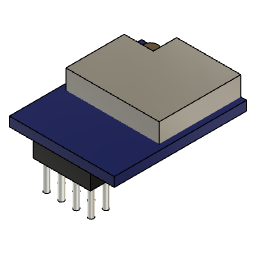
MLE21 v1.0 (Autodesk Fusion 360 archive; units mm, degrees)
design "RA-02"
Autodesk Fusion 360 part; units mm, degrees
sketch "Esquisse1" plane through (0, 0, 0) normal (0, 0, 1) x (1, 0, 0) in component "LoRa RA-02"
  line L0 (0, 0) -> (18, 0)
  line L1 (18, 0) -> (18, -22.7)
  line L2 (18, -22.7) -> (0, -22.7)
  line L3 (0, -22.7) -> (0, 0)
  line L4 (1, 0) -> (17, 0)
  line L5 (17, 0) -> (17, -14)
  line L6 (17, -14) -> (1, -14)
  line L7 (1, -14) -> (1, 0)
  line L8 (13.9, -22.7) -> (4.1, -22.7)
  line L9 (4.1, -22.7) -> (4.1, -17.7)
  line L10 (4.1, -17.7) -> (13.9, -17.7)
  line L11 (13.9, -17.7) -> (13.9, -22.7)
  line L12 (1, 0) -> (6, 0)
  line L13 (6, 0) -> (6, -4)
  line L14 (6, -4) -> (1, -4)
  line L15 (1, -4) -> (1, 0)
  circle A0 centre (3.5142, -2) radius 1.25
  circle A1 centre (5.2, -21.5) radius 0.445
  circle A2 centre (7.74, -21.5) radius 0.445
  circle A3 centre (10.28, -21.5) radius 0.445
  circle A4 centre (12.82, -21.5) radius 0.445
  circle A5 centre (5.2, -18.96) radius 0.445
  circle A6 centre (7.74, -18.96) radius 0.445
  circle A7 centre (10.28, -18.96) radius 0.445
  circle A8 centre (12.82, -18.96) radius 0.445
  dimension "d1" = 18
  dimension "d2" = 22.7
  dimension "d3" = 16
  dimension "d4" = 14
  dimension "d5" = 9.8
  dimension "d6" = 5
  dimension "d7" = 5
  dimension "d8" = 4
  dimension "d9" = 2.5
  dimension "d18" = 0.89
  dimension "d21" = 7.62
  dimension "d22" = 2.54
  dimension "d23" = 1.2
  dimension "d24" = 1.1
  constraint horizontal L0
  constraint vertical L1
  constraint horizontal L2
  constraint vertical L3
  constraint coincident L0.start L3.end
  constraint horizontal L4
  constraint vertical L5
  constraint horizontal L6
  constraint vertical L7
  constraint coincident L0 L4.start
  constraint midpoint L0 L4
  constraint horizontal L8
  constraint vertical L9
  constraint horizontal L10
  constraint vertical L11
  constraint coincident L2 L8.start
  constraint midpoint L2 L8
  constraint horizontal L12
  constraint vertical L13
  constraint horizontal L14
  constraint vertical L15
  measures "d1" distance of L0.start L0.end
  measures "d2" distance of L0.start L2.end
  measures "d3" distance of L4.start L4.end
  measures "d4" distance of L4.start L6.end
  measures "d5" distance of L8.start L8.end
  measures "d6" distance of L8.start L10.end
  measures "d7" distance of L4.start L12.end
  measures "d8" distance of L4.start L14.end
  measures "d9" diameter of A0
  measures "d18" diameter of A1
  measures "d23" distance of L2 A1.centre
  measures "d24" distance of L9 A1.centre
extrude "Extrusion1" add sketch "Esquisse1" along normal blind 1.6 contours L0 L1 L2 L3 L5 L6 L7 L9 L10 L11 L15 | L0 L4 L7 L12 L13 L14 L15 | L0 L4 L5 L6 L7 L13 L14 | L2 L8 L9 L10 L11 | A0 | A1 | A2 | A3 | A4 | A5 | A6 | A7 | A8 makes body 1 in component "LoRa RA-02"
extrude "Extrusion2" add sketch "Esquisse1" against normal blind 2.6 separate body contours L2 L8 L9 L10 L11 | A1 | A2 | A3 | A4 | A5 | A6 | A7 | A8 makes body 2 in component "LoRa RA-02"
extrude "Extrusion3" add sketch "Esquisse1" along normal blind 4.9 separate body contours L0 L4 L5 L6 L7 L13 L14 makes body 3 in component "LoRa RA-02"
extrude "Extrusion4" add sketch "Esquisse1" along normal blind 3 separate body contours A0 makes body 4 in component "LoRa RA-02"
extrude "Extrusion5" add sketch "Esquisse1" against normal blind 5 from surface at -2.6 separate body contours A1 | A2 | A3 | A4 | A5 | A6 | A7 | A8 makes body 5 at (10.077, -19.356, -4.2667) makes body 6 at (8.1712, -21.6098, -5.9333) makes body 7 at (12.617, -21.896, -4.2667) makes body 8 at (8.1712, -19.0698, -5.9333) makes body 9 at (12.617, -19.356, -4.2667) makes body 10 at (5.6312, -21.6098, -5.9333) makes body 11 at (10.077, -21.896, -4.2667) makes body 12 at (5.6312, -19.0698, -5.9333) in component "LoRa RA-02"
component "LoRa RA-02" placed x (1, 0, 0) y (0, 1, 0) z (0, 0, 1) at (0, 0, 0)
named bodies: "PCB", "connecteur", "SX11278", "IPX"

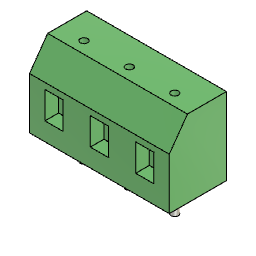
design "KF301-5.0-3P"
Autodesk Fusion 360 part; units mm, degrees
sketch "Esquisse1" plane through (0, 0, 0) normal (0, 0, 1) x (1, 0, 0) in component "KF128-2.54-2P"
  line L0 (0, 0) -> (15.4, 0)
  line L1 (15.4, 0) -> (15.4, 6.3)
  line L2 (15.4, 6.3) -> (0, 6.3)
  line L3 (0, 6.3) -> (0, 0)
  circle A0 centre (2.7, 3.3) radius 0.4
  circle A1 centre (7.7, 3.3) radius 0.4
  circle A2 centre (12.7, 3.3) radius 0.4
  dimension "d1" = 15.4
  dimension "d2" = 6.3
  dimension "d3" = 0.8
  dimension "d4" = 3
  dimension "d7" = 10
  dimension "d8" = 0
  dimension "d13" = 2.7
  constraint horizontal L0
  constraint vertical L1
  constraint horizontal L2
  constraint vertical L3
  constraint coincident L0.start L3.end
  measures "d1" distance of L0.start L0.end
  measures "d2" distance of L0.start L2.end
  measures "d3" diameter of A0
  measures "d4" distance of L2 A0.centre
  measures "d13" distance of L3 A0.centre
extrude "Extrusion1" add sketch "Esquisse1" along normal blind 8.5 makes body 1 in component "KF128-2.54-2P"
chamfer "Chanfrein1" distance 2 distance2 2.8333 1 edges at (7.7, 0, 8.5) measured on face at (7.69, 0.967, 8.5) on bodies 1 in component "KF128-2.54-2P"
sketch "Esquisse3" plane through (0, 0, 0) normal (0, -1, 0) x (1, 0, 0) in component "KF128-2.54-2P"
  line L0 (15.4, 5.6667) -> (0, 5.6667)
  line L1 (0, 5.6667) -> (0, 0)
  line L2 (0, 0) -> (15.4, 0)
  line L3 (15.4, 0) -> (15.4, 5.6667)
  line L4 (3.7, 5) -> (1.7, 5)
  line L5 (1.7, 5) -> (1.7, 2)
  line L6 (1.7, 2) -> (3.7, 2)
  line L7 (3.7, 2) -> (3.7, 5)
  line L8 (3.7, 5) -> (1.7, 2) construction
  line L9 (1.7, 5) -> (3.7, 2) construction
  line L10 (6.7, 2) -> (8.7, 2)
  line L11 (6.7, 5) -> (6.7, 2)
  line L12 (8.7, 5) -> (6.7, 5)
  line L13 (8.7, 2) -> (8.7, 5)
  line L14 (11.7, 2) -> (13.7, 2)
  line L15 (11.7, 5) -> (11.7, 2)
  line L16 (13.7, 5) -> (11.7, 5)
  line L17 (13.7, 2) -> (13.7, 5)
  point P0 (2.7, 3.5)
  dimension "d19" = 2
  dimension "d20" = 3
  dimension "d21" = 2.7
  dimension "d24" = 10
  dimension "d25" = 0
  constraint horizontal L4
  constraint perpendicular L4 L5
  constraint parallel L4 L6
  constraint parallel L5 L7
  constraint coincident L8 P0
  constraint coincident L9 P0
  measures "d19" distance of L5.end L6.end
  measures "d20" distance of L4.end L5.end
  measures "d21" distance of L1 P0
extrude "Extrusion2" cut sketch "Esquisse3" against normal blind 1.5 contours L4 L5 L6 L7 | L10 L11 L12 L13 | L14 L15 L16 L17 bodies 1 in component "KF128-2.54-2P"
extrude "Extrusion3" add sketch "Esquisse1" against normal blind 3 separate body contours A0 | A1 | A2 makes body 2 at (3.0995, 3.2801, -2) makes body 3 at (8.0995, 3.2801, -2) makes body 4 at (13.0995, 3.2801, -2) in component "KF128-2.54-2P"
component "KF128-2.54-2P" placed x (1, 0, 0) y (0, 1, 0) z (0, 0, 1) at (0, 0, 0)
equation "d1 = ( pas * 3 ) + marge_cote"
equation "d2 = profondeur"
equation "d4 = marge_arriere"
equation "d7 = pas * 2"
equation "marge_arriere = 3 mm"
equation "pas = 5.0 mm"
equation "marge_cote = 0.4 mm"
equation "profondeur = 6.3 mm"
equation "d13 = pas / 2 + marge_cote / 2"
equation "hauteur = 8.5 mm"
equation "d15 = hauteur"
equation "d18 = hauteur / 3"
equation "d21 = pas / 2 + marge_cote / 2"
equation "d24 = pas * 2"
equation "nbpin = 3 mm"

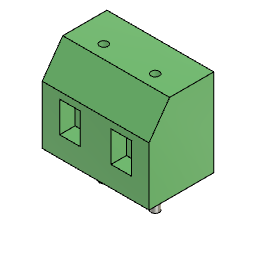
design "KF301-5.0-2P"
Autodesk Fusion 360 part; units mm, degrees
sketch "Esquisse1" plane through (0, 0, 0) normal (0, 0, 1) x (1, 0, 0) in component "KF128-2.54-2P"
  line L0 (0, 0) -> (10.4, 0)
  line L1 (10.4, 0) -> (10.4, 6.3)
  line L2 (10.4, 6.3) -> (0, 6.3)
  line L3 (0, 6.3) -> (0, 0)
  circle A0 centre (2.7, 3.3) radius 0.4
  circle A1 centre (7.7, 3.3) radius 0.4
  dimension "d1" = 10.4
  dimension "d2" = 6.3
  dimension "d3" = 0.8
  dimension "d4" = 3
  dimension "d7" = 5
  dimension "d8" = 0
  dimension "d13" = 2.7
  constraint horizontal L0
  constraint vertical L1
  constraint horizontal L2
  constraint vertical L3
  constraint coincident L0.start L3.end
  measures "d1" distance of L0.start L0.end
  measures "d2" distance of L0.start L2.end
  measures "d3" diameter of A0
  measures "d4" distance of L2 A0.centre
  measures "d13" distance of L3 A0.centre
extrude "Extrusion1" add sketch "Esquisse1" along normal blind 8.5 makes body 1 in component "KF128-2.54-2P"
chamfer "Chanfrein1" distance 2 distance2 2.8333 1 edges at (5.2, 0, 8.5) measured on face at (4.4154, 0.9759, 8.5) on bodies 1 in component "KF128-2.54-2P"
sketch "Esquisse3" plane through (0, 0, 0) normal (0, -1, 0) x (1, 0, 0) in component "KF128-2.54-2P"
  line L0 (10.4, 5.6667) -> (0, 5.6667)
  line L1 (0, 5.6667) -> (0, 0)
  line L2 (0, 0) -> (10.4, 0)
  line L3 (10.4, 0) -> (10.4, 5.6667)
  line L4 (3.7, 5) -> (1.7, 5)
  line L5 (1.7, 5) -> (1.7, 2)
  line L6 (1.7, 2) -> (3.7, 2)
  line L7 (3.7, 2) -> (3.7, 5)
  line L8 (3.7, 5) -> (1.7, 2) construction
  line L9 (1.7, 5) -> (3.7, 2) construction
  line L10 (6.7, 2) -> (8.7, 2)
  line L11 (6.7, 5) -> (6.7, 2)
  line L12 (8.7, 5) -> (6.7, 5)
  line L13 (8.7, 2) -> (8.7, 5)
  point P0 (2.7, 3.5)
  dimension "d19" = 2
  dimension "d20" = 3
  dimension "d21" = 2.7
  dimension "d24" = 5
  dimension "d25" = 0
  constraint horizontal L4
  constraint perpendicular L4 L5
  constraint parallel L4 L6
  constraint parallel L5 L7
  constraint coincident L8 P0
  constraint coincident L9 P0
  measures "d19" distance of L5.end L6.end
  measures "d20" distance of L4.end L5.end
  measures "d21" distance of L1 P0
extrude "Extrusion2" cut sketch "Esquisse3" against normal blind 1.5 contours L4 L5 L6 L7 | L10 L11 L12 L13 bodies 1 in component "KF128-2.54-2P"
extrude "Extrusion3" add sketch "Esquisse1" against normal blind 3 separate body contours A0 | A1 makes body 2 at (3.0995, 3.2801, -2) makes body 3 at (8.0995, 3.2801, -2) in component "KF128-2.54-2P"
component "KF128-2.54-2P" placed x (1, 0, 0) y (0, 1, 0) z (0, 0, 1) at (0, 0, 0)
equation "d1 = ( pas * 2 ) + marge_cote"
equation "d2 = profondeur"
equation "d4 = marge_arriere"
equation "d7 = pas"
equation "marge_arriere = 3 mm"
equation "pas = 5.0 mm"
equation "marge_cote = 0.4 mm"
equation "profondeur = 6.3 mm"
equation "d13 = pas / 2 + marge_cote / 2"
equation "hauteur = 8.5 mm"
equation "d15 = hauteur"
equation "d18 = hauteur / 3"
equation "d21 = pas / 2 + marge_cote / 2"
equation "d24 = pas"
